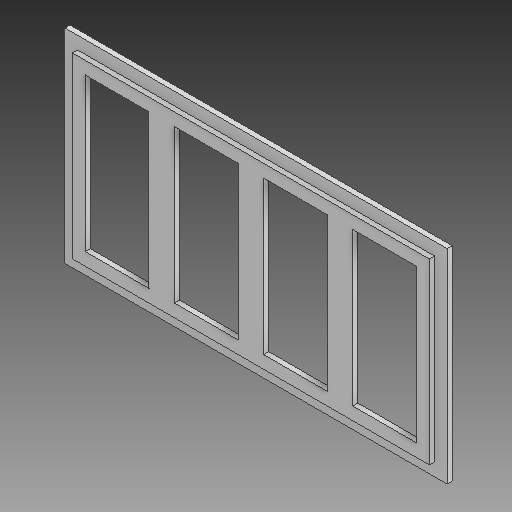
# Autodesk Inventor part: Belüftung
Saved by Autodesk Inventor 2021 (Build 250183000, 183)
## iProperties
Created: 2021-11-19
Part Number: Belüftung
Material: Generisch
Document SubType Name: Modeling
Designer: lukas
Density: 1 g/cm^3
Appearance: Vorgabe
Stock Number: Belüftung
Author: lukas
Autodesk Inventor part; units mm, degrees
ref_plane "YZ Plane" through (0, 0, 0) normal (1, 0, 0) x (0, 1, 0)
ref_plane "XZ Plane" through (0, 0, 0) normal (0, 1, 0) x (-1, 0, 0)
ref_plane "XY Plane" through (0, 0, 0) normal (0, 0, 1) x (1, 0, 0)
sketch "Skizze1" plane through (0, 0, 0) normal (0, 0, 1) x (1, 0, 0)
  line L0 (0, -78.9916) -> (0, 33.0084) projected
  line L1 (-75, 17.0084) -> (75, 17.0084)
  line L2 (75, 17.0084) -> (75, -62.9916)
  line L3 (75, -62.9916) -> (-75, -62.9916)
  line L4 (-75, -62.9916) -> (-75, 17.0084)
  point P0 (0, 0)
  dimension "d0" = 150
  dimension "d1" = 80
  constraints: 8 end point, 2 parallel, 1 horizontal, 1 perpendicular, 1 other
  measures "d0" distance of L2.end L3.end
  measures "d1" distance between parallel lines of L1 L3
extrude "Extrusion1" add sketch "Skizze1" along normal blind 2
sketch "Skizze2" plane through (0, 0, 2) normal (0, 0, 1) x (1, 0, 0)
  line L0 (-70, 12.0084) -> (70, 12.0084)
  line L1 (70, 12.0084) -> (70, -57.9916)
  line L2 (70, -57.9916) -> (-70, -57.9916)
  line L3 (-70, -57.9916) -> (-70, 12.0084)
  line L4 (75, 17.0084) -> (-75, 17.0084) projected
  line L5 (75, -62.9916) -> (75, 17.0084) projected
  point P0 (0, 0)
  dimension "d4" = 70
  dimension "d5" = 140
  dimension "d6" = 5
  dimension "d7" = 5
  constraints: 8 end point, 2 parallel, 1 horizontal, 1 perpendicular
  measures "d4" distance between parallel lines of L2 L0
  measures "d5" distance between parallel lines of L1 L3
  measures "d6" distance between parallel lines of L4 L0
  measures "d7" distance between parallel lines of L5 L1
extrude "Extrusion2" add sketch "Skizze2" along normal blind 2
sketch "Skizze3" plane through (0, 0, 4) normal (0, 0, 1) x (1, 0, 0)
  line L0 (70, 12.0084) -> (-70, 12.0084) projected
  line L1 (-40, 12.0084) -> (-40, -57.9916)
  line L2 (-40, -57.9916) -> (-30, -57.9916)
  line L3 (-70, -57.9916) -> (70, -57.9916) projected
  line L4 (-40, 12.0084) -> (-30, 12.0084)
  line L5 (-30, 12.0084) -> (-30, -57.9916)
  line L6 (-5, -57.9916) -> (5, -57.9916)
  line L7 (5, -57.9916) -> (5, 12.0084)
  line L8 (5, 12.0084) -> (-5, 12.0084)
  line L9 (-5, 12.0084) -> (-5, -57.9916)
  line L10 (39.912, -57.9916) -> (40, -57.9916)
  line L11 (40, -57.9916) -> (40, 12.0084)
  line L12 (40, 12.0084) -> (30, 12.0084)
  line L13 (30, 12.0084) -> (30, -57.9916)
  line L14 (-70, 12.0084) -> (-70, -57.9916) projected
  line L15 (70, -57.9916) -> (70, 12.0084) projected
  line L16 (30, -57.9916) -> (40, -57.9916)
  line L17 (40, 7.0084) -> (65, 7.0084)
  line L18 (65, 7.0084) -> (65, -52.9916)
  line L19 (65, -52.9916) -> (40, -52.9916)
  line L20 (-40, 7.0084) -> (-65, 7.0084)
  line L21 (-65, 7.0084) -> (-65, -52.9916)
  line L22 (-65, -52.9916) -> (-40, -52.9916)
  line L23 (-40, 7.0084) -> (40, 7.0084)
  line L24 (-40, -52.9916) -> (40, -52.9916)
  point P0 (0, 0)
  point P1 (5, -52.9916)
  point P2 (30, -52.9916)
  point P3 (30, 7.0084)
  point P4 (5, 7.0084)
  point P5 (-30, -52.9916)
  point P6 (-5, -52.9916)
  point P7 (-5, 7.0084)
  point P8 (-30, 7.0084)
  dimension "d12" = 10
  dimension "d13" = 10
  dimension "d14" = 10
  dimension "d15" = 30
  dimension "d16" = 30
  dimension "d17" = 25
  dimension "d18" = 5
  dimension "d19" = 5
  dimension "d20" = 5
  dimension "d21" = 5
  dimension "d22" = 5
  dimension "d23" = 5
  constraints: 42 end point, 15 point on line, 11 perpendicular, 2 horizontal, 1 collinear
  measures "d12" distance between parallel lines of L5 L1
  measures "d13" distance between parallel lines of L7 L9
  measures "d14" distance between parallel lines of L11 L13
  measures "d15" distance between parallel lines of L1 L14
  measures "d16" distance between parallel lines of L11 L15
  measures "d17" distance between parallel lines of L9 L5
  measures "d18" distance between parallel lines of L19 L3
  measures "d19" distance between parallel lines of L15 L18
  measures "d20" distance between parallel lines of L0 L17
  measures "d21" distance between parallel lines of L21 L14
  measures "d22" distance between parallel lines of L22 L3
  measures "d23" distance between parallel lines of L0 L20
extrude "Extrusion3" cut sketch "Skizze3" against normal blind 5 contours L17 L18 L19 L11 | L13 L24 L7 L23 | L9 L24 L5 L23 | L1 L22 L21 L20
sketch "Skizze4" plane through (0, 0, 0) normal (0, 0, -1) x (-1, 0, 0)
  line L0 (-70, -57.9916) -> (-70, 12.0084) projected
  line L1 (70, 12.0084) -> (70, -57.9916) projected
  line L2 (-70, 12.0084) -> (70, 12.0084)
  line L3 (70, 12.0084) -> (70, -57.9916)
  line L4 (70, -57.9916) -> (-70, -57.9916)
  line L5 (-70, -57.9916) -> (-70, 12.0084)
  point P0 (0, 0)
  constraints: 8 end point, 2 parallel, 1 horizontal, 1 perpendicular
extrude "Extrusion4" cut sketch "Skizze4" against normal blind 2
